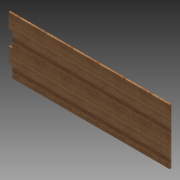
# Autodesk Inventor part: manipulator side pannel 2
Saved by Autodesk Inventor 2012 (Build 160160000, 160)
## iProperties
Created: 2013-09-02
Part Number: manipulator side pannel 2
Material: Default
Document SubType Name: Modeling
Designer: Bryce
Density: 1 g/cm^3
Author: Bryce
Autodesk Inventor part; units mm, degrees
ref_plane "YZ Plane" through (0, 0, 0) normal (1, 0, 0) x (0, 1, 0)
ref_plane "XZ Plane" through (0, 0, 0) normal (0, 1, 0) x (-1, 0, 0)
ref_plane "XY Plane" through (0, 0, 0) normal (0, 0, 1) x (1, 0, 0)
sketch "Sketch1" plane through (0, 0, 0) normal (0, 0, 1) x (1, 0, 0)
  line L0 (0, 0) -> (539.75, 0)
  line L1 (539.75, 0) -> (539.75, 190.5)
  line L2 (539.75, 190.5) -> (0, 190.5)
  line L3 (0, 38.1) -> (-12.7, 38.1)
  line L4 (-12.7, 38.1) -> (-12.7, 88.9)
  line L5 (-12.7, 88.9) -> (0, 88.9)
  line L6 (0, 190.5) -> (-12.7, 190.5)
  line L7 (-12.7, 190.5) -> (-12.7, 139.7)
  line L8 (-12.7, 139.7) -> (0, 139.7)
  line L9 (0, 139.7) -> (0, 190.5) construction
  line L10 (0, 139.7) -> (0, 88.9)
  line L11 (0, 88.9) -> (0, 38.1) construction
  line L12 (0, 38.1) -> (0, 0)
  dimension "d0" = 190.5
  dimension "d1" = 539.75
  dimension "d10" = 12.7
  dimension "d11" = 50.8
  dimension "d12" = 50.8
  dimension "d13" = 50.8
  constraints: 26 end point, 8 parallel, 3 horizontal, 3 perpendicular, 1 point on line
  measures "d0" distance of L2.end L0.start
  measures "d1" distance of L1.end L2.end
  measures "d10" distance of L2.end L6.end
  measures "d11" distance of L6.end L7.end
  measures "d12" distance of L3.end L4.end
  measures "d13" distance between parallel lines of L8 L5
extrude "Extrusion1" add sketch "Sketch1" against normal blind 6.35
body "Solid1"
